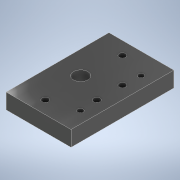
# Autodesk Inventor part: tapaperfil
Saved by Autodesk Inventor 2022 (Build 260153000, 153)
## iProperties
Created: 2022-03-21
Part Number: tapaperfil
Material: Generic
Document SubType Name: Modeling
Designer: ferna
Density: 1 g/cm^3
Appearance: Dark Gray
Mass: 45.8288 g
Surface Area: 124.801 cm^2
Volume: 45.8288 cm^3
Author: ferna
Autodesk Inventor part; units mm, degrees
ref_plane "YZ Plane" through (0, 0, 0) normal (1, 0, 0) x (0, 1, 0)
ref_plane "XZ Plane" through (0, 0, 0) normal (0, 1, 0) x (-1, 0, 0)
ref_plane "XY Plane" through (0, 0, 0) normal (0, 0, 1) x (1, 0, 0)
sketch "Sketch1" plane through (0, 0, 0) normal (0, 1, 0) x (-1, 0, 0)
  line L0 (0, 0) -> (50.5, 0)
  line L1 (50.5, 0) -> (50.5, -80)
  line L2 (50.5, -80) -> (0, -80)
  line L3 (0, -80) -> (0, 0)
  line L4 (0, -80) -> (9.1, -80)
  line L5 (0, -80) -> (10, -80)
  line L6 (10, -80) -> (10, -50)
  circle A0 centre (10, -30) radius 2.5
  circle A1 centre (10, -50) radius 2.5
  line L7 (9.1, -65.7) -> (9.1, -63.6)
  circle A2 centre (9.1, -16.4) radius 2.1
  circle A3 centre (9.1, -63.6) radius 2.1
  line L8 (0, 0) -> (0, -40)
  line L9 (9.1, -40) -> (32.5, -40)
  circle A4 centre (32.5, -40) radius 5.6
  line L10 (0, 0) -> (0, -10)
  line L11 (30, -10) -> (30, -70)
  circle A5 centre (30, -10) radius 2.5
  circle A6 centre (30, -70) radius 2.5
  line L12 (27.5, -10) -> (30, -10)
  line L13 (9.1, 0) -> (9.1, -10)
  line L14 (9.1, -14.3) -> (9.1, -16.4)
  line L15 (9.1, -10) -> (9.1, 0)
  line L16 (9.1, -18.5) -> (9.1, -14.3)
  line L17 (10, -18.2974) -> (10, -14.5026)
  line L18 (10, -50) -> (10, -47.5)
  line L19 (10, -32.5) -> (10, -30)
  line L20 (9.1, -32.3324) -> (9.1, -27.6676)
  line L21 (10, -80) -> (10, -47.5)
  line L22 (10, -40) -> (10, -27.5)
  line L23 (9.1, -65.7) -> (9.1, -61.5)
  line L24 (9.1, -52.3324) -> (9.1, -47.6676)
  dimension "d17" = 5
  dimension "d0" = 50.5
  dimension "d1" = 80
  dimension "d2" = 9.1
  dimension "d3" = 10
  dimension "d4" = 30
  dimension "d5" = 20
  dimension "d6" = 5
  dimension "d7" = 5
  dimension "d8" = 16.4
  dimension "d9" = 16.4
  dimension "d10" = 4.2
  dimension "d11" = 4.2
  dimension "d12" = 32.5
  dimension "d13" = 11.2
  dimension "d14" = 10
  dimension "d15" = 30
  dimension "d16" = 60
  dimension "d27" = 47.2
  constraints: 50 end point, 13 point on circle, 12 perpendicular, 7 coincident, 7 point on line, 6 centre point, 3 midpoint, 2 parallel, 1 horizontal, 1 horizontal alignment, 2 other
  measures "d0" distance of L1.end L2.end
  measures "d1" distance of L0.end L1.end
  measures "d2" distance of L2.end L4.end
  measures "d3" distance of L2.end L5.end
  measures "d4" distance of L5.end L6.end
  measures "d5" distance of L6.end L19.end
  measures "d6" diameter of A0
  measures "d7" diameter of A1
  measures "d8" distance of L4.end L7.end
  measures "d9" distance of L13.start L14.end
  measures "d10" diameter of A2
  measures "d11" diameter of A3
  measures "d12" distance of L8.end L9.end
  measures "d13" diameter of A4
  measures "d14" distance of L0.start L10.end
  measures "d15" distance of L10.end L11.start
  measures "d16" distance of L11.start L11.end
  measures "d27" distance of L14.end L7.end
extrude "Extrusion1" add sketch "Sketch1" along normal blind 12
sketch "Sketch2" plane through (-50.5, 0, -80) normal (-1, 0, 0) x (0, 0, 1)
  line L0 (80, 0) -> (80, 12) projected
  line L1 (80, 0) -> (40, 0)
  line L2 (0, 0) -> (80, 0) projected
  line L3 (40, 0) -> (49.9, 0)
  line L4 (49.9, 0) -> (30.1, 0)
  line L5 (30.1, 0) -> (30.1, 6)
  line L6 (30.1, 6) -> (49.9, 6)
  circle A0 centre (49.9, 6) radius 2.1
  circle A1 centre (30.1, 6) radius 2.1
  dimension "d20" = 9.9
  dimension "d21" = 19.8
  dimension "d22" = 6
  dimension "d23" = 4.2
  dimension "d24" = 4.2
  constraints: 10 end point, 2 centre point, 2 coincident, 2 perpendicular, 2 point on line, 1 midpoint
  measures "d20" distance of L1.end L3.end
  measures "d21" distance of L3.end L4.end
  measures "d22" distance of L4.end L5.end
  measures "d23" diameter of A0
  measures "d24" diameter of A1
extrude "Extrusion2" cut sketch "Sketch2" against normal blind 7
sketch "Sketch3" plane through (-50.5, 0, -80) normal (-1, 0, 0) x (0, 0, 1)
  circle A0 centre (30.1, 6) radius 2.1 projected
  circle A1 centre (49.9, 6) radius 2.1 projected
  line L0 (0, 0) -> (80, 0) projected
  line L1 (80, 0) -> (80, 12) projected
  line L2 (0, 12) -> (80, 12) projected
  line L3 (0, 0) -> (0, 12) projected
body "Solid1"
